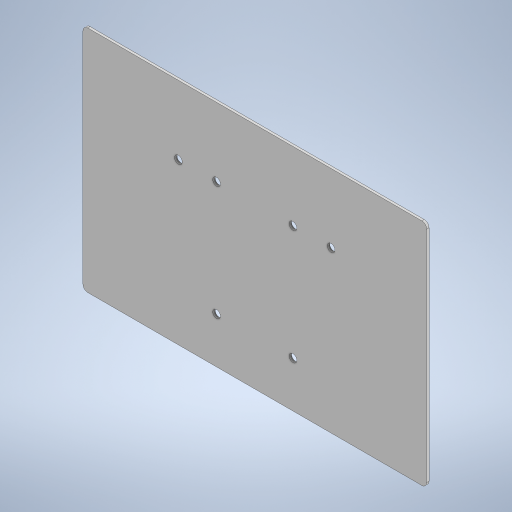
# Autodesk Inventor part: Kicker poly
Saved by Autodesk Inventor 2023 (Build 270158000, 158)
## iProperties
Created: 2024-02-16
Part Number: Kicker poly
Material: Generic
Document SubType Name: Modeling
Designer: Robodox
Density: 1 g/cm^3
Appearance: Default
Author: Robodox
Autodesk Inventor part; units mm, degrees
ref_plane "YZ Plane" through (0, 0, 0) normal (1, 0, 0) x (0, 1, 0)
ref_plane "XZ Plane" through (0, 0, 0) normal (0, 1, 0) x (-1, 0, 0)
ref_plane "XY Plane" through (0, 0, 0) normal (0, 0, 1) x (1, 0, 0)
sketch "Sketch1" plane through (0, 0, 0) normal (0, 0, 1) x (1, 0, 0)
  line L0 (0, 0) -> (228.6, 0)
  line L1 (228.6, 0) -> (228.6, 152.4)
  line L2 (228.6, 152.4) -> (0, 152.4)
  line L3 (0, 152.4) -> (0, 0)
  line L4 (0, 152.4) -> (50.8, 152.4)
  line L5 (50.8, 152.4) -> (50.8, 0)
  line L6 (228.6, 152.4) -> (177.8, 152.4)
  line L7 (177.8, 152.4) -> (177.8, 0)
  line L8 (50.8, 0) -> (50.8, 30.48)
  line L9 (50.8, 30.48) -> (88.9, 30.48)
  circle A0 centre (88.9, 30.48) radius 2.54
  line L10 (88.9, 30.48) -> (139.7, 30.48)
  circle A1 centre (139.7, 30.48) radius 2.54
  line L11 (139.7, 30.48) -> (139.7, 106.68)
  circle A2 centre (139.7, 106.68) radius 2.54
  line L12 (88.9, 30.48) -> (88.9, 106.68)
  circle A3 centre (88.9, 106.68) radius 2.54
  line L13 (88.9, 106.68) -> (139.7, 106.68)
  line L14 (139.7, 106.68) -> (165.1, 106.68)
  circle A4 centre (165.1, 106.68) radius 2.54
  line L15 (88.9, 106.68) -> (63.5, 106.68)
  circle A5 centre (63.5, 106.68) radius 2.54
  dimension "d0" = 228.6
  dimension "d1" = 152.4
  dimension "d2" = 50.8
  dimension "d3" = 50.8
  dimension "d4" = 30.48
  dimension "d5" = 38.1
  dimension "d6" = 5.08
  dimension "d7" = 50.8
  dimension "d8" = 5.08
  dimension "d9" = 76.2
  dimension "d10" = 5.08
  dimension "d11" = 5.08
  dimension "d12" = 25.4
  dimension "d13" = 5.08
  dimension "d14" = 25.4
  dimension "d15" = 5.08
  constraints: 32 end point, 7 perpendicular, 6 centre point, 6 coincident, 5 horizontal, 5 point on line, 1 vertical
  measures "d0" distance of L0.start L0.end
  measures "d1" distance of L0.end L1.end
  measures "d2" distance of L2.end L4.end
  measures "d3" distance of L1.end L6.end
  measures "d4" distance of L5.end L8.end
  measures "d5" distance of L8.end L9.end
  measures "d6" diameter of A0
  measures "d7" distance of L10.start L10.end
  measures "d8" diameter of A1
  measures "d9" distance of L11.start L11.end
  measures "d10" diameter of A2
  measures "d11" diameter of A3
  measures "d12" distance of L13.end L14.end
  measures "d13" diameter of A4
  measures "d14" distance of L13.start L15.end
  measures "d15" diameter of A5
extrude "Extrusion1" add sketch "Sketch1" along normal blind 1.5875 contours L3 L2 L5 L0 | L5 L2 L7 L0 | L7 L2 L1 L0 | L12 A3 L13 A2 L11 A1 L10 A0
fillet "Fillet1" radius 3.175 4 edges at (0, 152.4, 0.7937) (228.6, 152.4, 0.7937) (228.6, 0, 0.7937) (0, 0, 0.7937)
body "Solid1"
